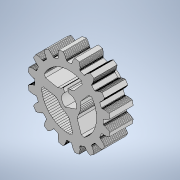
# Autodesk Inventor part: Ведущая шестерня дифференециала
Saved by Autodesk Inventor 2020 (Build 240168000, 168)
## iProperties
Created: 2021-05-23
Part Number: Ведущая шестерня дифференециала
Material: Типовые
Document SubType Name: Modeling
Designer: Антон
Density: 1 g/cm^3
Appearance: По умолчанию
Author: Антон
Autodesk Inventor part; units mm, degrees
(part 1 of 2)
ref_plane "YZ Plane" through (0, 0, 0) normal (1, 0, 0) x (0, 1, 0)
ref_plane "XZ Plane" through (0, 0, 0) normal (0, 1, 0) x (-1, 0, 0)
ref_plane "XY Plane" through (0, 0, 0) normal (0, 0, 1) x (1, 0, 0)
sketch "Эскиз1" plane through (0, 0, 0) normal (0, 0, 1) x (1, 0, 0)
  line L0 (1.5404, 9.3026) -> (1.5076, 9.387)
  line L1 (1.5076, 9.387) -> (1.4717, 9.4203)
  line L2 (1.4717, 9.4203) -> (1.4352, 9.4443)
  line L3 (1.4352, 9.4443) -> (1.3612, 9.4785)
  line L4 (1.3612, 9.4785) -> (1.2865, 9.5017)
  line L5 (1.2865, 9.5017) -> (1.2112, 9.5182)
  line L6 (1.2112, 9.5182) -> (1.0615, 9.5608)
  line L7 (1.0615, 9.5608) -> (0.9133, 9.6174)
  line L8 (0.9133, 9.6174) -> (0.7663, 9.6852)
  line L9 (0.7663, 9.6852) -> (0.6208, 9.7626)
  line L10 (0.6208, 9.7626) -> (0.4767, 9.8489)
  line L11 (0.4767, 9.8489) -> (0.3343, 9.9435)
  line L12 (0.3343, 9.9435) -> (0.1935, 10.0459)
  line L13 (0.1935, 10.0459) -> (0.0892, 10.1277)
  line L14 (0.0892, 10.1277) -> (0.2775, 11.074)
  line L15 (0.2775, 11.074) -> (0.4052, 11.1097)
  line L16 (0.4052, 11.1097) -> (0.5744, 11.1505)
  line L17 (0.5744, 11.1505) -> (0.7422, 11.1834)
  line L18 (0.7422, 11.1834) -> (0.9083, 11.208)
  line L19 (0.9083, 11.208) -> (1.0724, 11.2238)
  line L20 (1.0724, 11.2238) -> (1.2341, 11.2302)
  line L21 (1.2341, 11.2302) -> (1.3927, 11.2258)
  line L22 (1.3927, 11.2258) -> (1.5473, 11.2079)
  line L23 (1.5473, 11.2079) -> (1.6232, 11.1943)
  line L24 (1.6232, 11.1943) -> (1.7011, 11.1871)
  line L25 (1.7011, 11.1871) -> (1.7825, 11.1904)
  line L26 (1.7825, 11.1904) -> (1.8254, 11.1986)
  line L27 (1.8254, 11.1986) -> (1.8713, 11.2156)
  line L28 (1.8713, 11.2156) -> (1.9339, 11.281)
  line L29 (1.9339, 11.281) -> (2.2631, 12.0757)
  line L30 (2.2631, 12.0757) -> (2.2651, 12.1663)
  line L31 (2.2651, 12.1663) -> (2.2447, 12.2108)
  line L32 (2.2447, 12.2108) -> (2.2201, 12.247)
  line L33 (2.2201, 12.247) -> (2.1649, 12.3068)
  line L34 (2.1649, 12.3068) -> (2.1047, 12.3569)
  line L35 (2.1047, 12.3569) -> (2.0415, 12.4009)
  line L36 (2.0415, 12.4009) -> (1.9195, 12.4975)
  line L37 (1.9195, 12.4975) -> (1.8042, 12.6066)
  line L38 (1.8042, 12.6066) -> (1.6944, 12.7254)
  line L39 (1.6944, 12.7254) -> (1.5896, 12.8527)
  line L40 (1.5896, 12.8527) -> (1.4895, 12.9875)
  line L41 (1.4895, 12.9875) -> (1.3941, 13.1294)
  line L42 (1.3941, 13.1294) -> (1.3032, 13.2779)
  line L43 (1.3032, 13.2779) -> (1.2382, 13.3934)
  line L44 (1.2382, 13.3934) -> (1.7742, 14.1957)
  line L45 (1.7742, 14.1957) -> (1.9058, 14.1797)
  line L46 (1.9058, 14.1797) -> (2.0778, 14.1527)
  line L47 (2.0778, 14.1527) -> (2.2454, 14.1188)
  line L48 (2.2454, 14.1188) -> (2.4083, 14.078)
  line L49 (2.4083, 14.078) -> (2.5659, 14.0298)
  line L50 (2.5659, 14.0298) -> (2.7177, 13.9738)
  line L51 (2.7177, 13.9738) -> (2.8626, 13.909)
  line L52 (2.8626, 13.909) -> (2.9986, 13.8333)
  line L53 (2.9986, 13.8333) -> (3.0635, 13.7917)
  line L54 (3.0635, 13.7917) -> (3.1327, 13.7553)
  line L55 (3.1327, 13.7553) -> (3.2092, 13.7272)
  line L56 (3.2092, 13.7272) -> (3.2519, 13.7183)
  line L57 (3.2519, 13.7183) -> (3.3009, 13.7165)
  line L58 (3.3009, 13.7165) -> (3.3838, 13.753)
  line L59 (3.3838, 13.753) -> (3.9921, 14.3612)
  line L60 (3.9921, 14.3612) -> (4.0285, 14.4441)
  line L61 (4.0285, 14.4441) -> (4.0267, 14.4931)
  line L62 (4.0267, 14.4931) -> (4.0179, 14.5359)
  line L63 (4.0179, 14.5359) -> (3.9898, 14.6123)
  line L64 (3.9898, 14.6123) -> (3.9533, 14.6815)
  line L65 (3.9533, 14.6815) -> (3.9117, 14.7464)
  line L66 (3.9117, 14.7464) -> (3.836, 14.8824)
  line L67 (3.836, 14.8824) -> (3.7712, 15.0273)
  line L68 (3.7712, 15.0273) -> (3.7152, 15.1791)
  line L69 (3.7152, 15.1791) -> (3.6671, 15.3368)
  line L70 (3.6671, 15.3368) -> (3.6262, 15.4996)
  line L71 (3.6262, 15.4996) -> (3.5924, 15.6672)
  line L72 (3.5924, 15.6672) -> (3.5653, 15.8392)
  line L73 (3.5653, 15.8392) -> (3.5494, 15.9708)
  line L74 (3.5494, 15.9708) -> (4.3516, 16.5068)
  line L75 (4.3516, 16.5068) -> (4.4671, 16.4418)
  line L76 (4.4671, 16.4418) -> (4.6156, 16.351)
  line L77 (4.6156, 16.351) -> (4.7575, 16.2555)
  line L78 (4.7575, 16.2555) -> (4.8924, 16.1555)
  line L79 (4.8924, 16.1555) -> (5.0196, 16.0506)
  line L80 (5.0196, 16.0506) -> (5.1384, 15.9408)
  line L81 (5.1384, 15.9408) -> (5.2475, 15.8255)
  line L82 (5.2475, 15.8255) -> (5.3441, 15.7035)
  line L83 (5.3441, 15.7035) -> (5.3882, 15.6403)
  line L84 (5.3882, 15.6403) -> (5.4382, 15.5801)
  line L85 (5.4382, 15.5801) -> (5.4981, 15.5249)
  line L86 (5.4981, 15.5249) -> (5.5342, 15.5004)
  line L87 (5.5342, 15.5004) -> (5.5787, 15.4799)
  line L88 (5.5787, 15.4799) -> (5.6693, 15.4819)
  line L89 (5.6693, 15.4819) -> (6.464, 15.8111)
  line L90 (6.464, 15.8111) -> (6.5294, 15.8737)
  line L91 (6.5294, 15.8737) -> (6.5464, 15.9196)
  line L92 (6.5464, 15.9196) -> (6.5547, 15.9626)
  line L93 (6.5547, 15.9626) -> (6.5579, 16.0439)
  line L94 (6.5579, 16.0439) -> (6.5508, 16.1219)
  line L95 (6.5508, 16.1219) -> (6.5372, 16.1977)
  line L96 (6.5372, 16.1977) -> (6.5193, 16.3523)
  line L97 (6.5193, 16.3523) -> (6.5149, 16.511)
  line L98 (6.5149, 16.511) -> (6.5212, 16.6726)
  line L99 (6.5212, 16.6726) -> (6.5371, 16.8367)
  line L100 (6.5371, 16.8367) -> (6.5617, 17.0028)
  line L101 (6.5617, 17.0028) -> (6.5945, 17.1706)
  line L102 (6.5945, 17.1706) -> (6.6353, 17.3399)
  line L103 (6.6353, 17.3399) -> (6.671, 17.4675)
  line L104 (6.671, 17.4675) -> (7.6173, 17.6558)
  line L105 (7.6173, 17.6558) -> (7.6991, 17.5515)
  line L106 (7.6991, 17.5515) -> (7.8015, 17.4107)
  line L107 (7.8015, 17.4107) -> (7.8961, 17.2683)
  line L108 (7.8961, 17.2683) -> (7.9824, 17.1242)
  line L109 (7.9824, 17.1242) -> (8.0598, 16.9787)
  line L110 (8.0598, 16.9787) -> (8.1276, 16.8317)
  line L111 (8.1276, 16.8317) -> (8.1842, 16.6835)
  line L112 (8.1842, 16.6835) -> (8.2268, 16.5338)
  line L113 (8.2268, 16.5338) -> (8.2433, 16.4585)
  line L114 (8.2433, 16.4585) -> (8.2665, 16.3838)
  line L115 (8.2665, 16.3838) -> (8.3007, 16.3099)
  line L116 (8.3007, 16.3099) -> (8.3247, 16.2734)
  line L117 (8.3247, 16.2734) -> (8.358, 16.2375)
  line L118 (8.358, 16.2375) -> (8.4424, 16.2046)
  line L119 (8.4424, 16.2046) -> (9.3026, 16.2046)
  line L120 (9.3026, 16.2046) -> (9.387, 16.2375)
  line L121 (9.387, 16.2375) -> (9.4203, 16.2734)
  line L122 (9.4203, 16.2734) -> (9.4443, 16.3099)
  line L123 (9.4443, 16.3099) -> (9.4785, 16.3838)
  line L124 (9.4785, 16.3838) -> (9.5017, 16.4585)
  line L125 (9.5017, 16.4585) -> (9.5182, 16.5338)
  line L126 (9.5182, 16.5338) -> (9.5608, 16.6835)
  line L127 (9.5608, 16.6835) -> (9.6174, 16.8317)
  line L128 (9.6174, 16.8317) -> (9.6852, 16.9787)
  line L129 (9.6852, 16.9787) -> (9.7626, 17.1242)
  line L130 (9.7626, 17.1242) -> (9.8489, 17.2683)
  line L131 (9.8489, 17.2683) -> (9.9435, 17.4107)
  line L132 (9.9435, 17.4107) -> (10.0459, 17.5515)
  line L133 (10.0459, 17.5515) -> (10.1277, 17.6558)
  line L134 (10.1277, 17.6558) -> (11.074, 17.4675)
  line L135 (11.074, 17.4675) -> (11.1097, 17.3399)
  line L136 (11.1097, 17.3399) -> (11.1505, 17.1706)
  line L137 (11.1505, 17.1706) -> (11.1834, 17.0028)
  line L138 (11.1834, 17.0028) -> (11.208, 16.8367)
  line L139 (11.208, 16.8367) -> (11.2238, 16.6726)
  line L140 (11.2238, 16.6726) -> (11.2302, 16.511)
  line L141 (11.2302, 16.511) -> (11.2258, 16.3523)
  line L142 (11.2258, 16.3523) -> (11.2079, 16.1977)
  line L143 (11.2079, 16.1977) -> (11.1943, 16.1219)
  line L144 (11.1943, 16.1219) -> (11.1871, 16.0439)
  line L145 (11.1871, 16.0439) -> (11.1904, 15.9626)
  line L146 (11.1904, 15.9626) -> (11.1986, 15.9196)
  line L147 (11.1986, 15.9196) -> (11.2156, 15.8737)
  line L148 (11.2156, 15.8737) -> (11.281, 15.8111)
  line L149 (11.281, 15.8111) -> (12.0757, 15.4819)
  line L150 (12.0757, 15.4819) -> (12.1663, 15.4799)
  line L151 (12.1663, 15.4799) -> (12.2108, 15.5004)
  line L152 (12.2108, 15.5004) -> (12.247, 15.5249)
  line L153 (12.247, 15.5249) -> (12.3068, 15.5801)
  line L154 (12.3068, 15.5801) -> (12.3569, 15.6403)
  line L155 (12.3569, 15.6403) -> (12.4009, 15.7035)
  line L156 (12.4009, 15.7035) -> (12.4975, 15.8255)
  line L157 (12.4975, 15.8255) -> (12.6066, 15.9408)
  line L158 (12.6066, 15.9408) -> (12.7254, 16.0506)
  line L159 (12.7254, 16.0506) -> (12.8527, 16.1555)
  line L160 (12.8527, 16.1555) -> (12.9875, 16.2555)
  line L161 (12.9875, 16.2555) -> (13.1294, 16.351)
  line L162 (13.1294, 16.351) -> (13.2779, 16.4418)
  line L163 (13.2779, 16.4418) -> (13.3934, 16.5068)
  line L164 (13.3934, 16.5068) -> (14.1957, 15.9708)
  line L165 (14.1957, 15.9708) -> (14.1797, 15.8392)
  line L166 (14.1797, 15.8392) -> (14.1527, 15.6672)
  line L167 (14.1527, 15.6672) -> (14.1188, 15.4996)
  line L168 (14.1188, 15.4996) -> (14.078, 15.3368)
  line L169 (14.078, 15.3368) -> (14.0298, 15.1791)
  line L170 (14.0298, 15.1791) -> (13.9738, 15.0273)
  line L171 (13.9738, 15.0273) -> (13.909, 14.8824)
  line L172 (13.909, 14.8824) -> (13.8333, 14.7464)
  line L173 (13.8333, 14.7464) -> (13.7917, 14.6815)
  line L174 (13.7917, 14.6815) -> (13.7553, 14.6123)
  line L175 (13.7553, 14.6123) -> (13.7272, 14.5359)
  line L176 (13.7272, 14.5359) -> (13.7183, 14.4931)
  line L177 (13.7183, 14.4931) -> (13.7165, 14.4441)
  line L178 (13.7165, 14.4441) -> (13.753, 14.3612)
  line L179 (13.753, 14.3612) -> (14.3612, 13.753)
  line L180 (14.3612, 13.753) -> (14.4441, 13.7165)
  line L181 (14.4441, 13.7165) -> (14.4931, 13.7183)
  line L182 (14.4931, 13.7183) -> (14.5359, 13.7272)
  line L183 (14.5359, 13.7272) -> (14.6123, 13.7553)
  line L184 (14.6123, 13.7553) -> (14.6815, 13.7917)
  line L185 (14.6815, 13.7917) -> (14.7464, 13.8333)
  line L186 (14.7464, 13.8333) -> (14.8824, 13.909)
  line L187 (14.8824, 13.909) -> (15.0273, 13.9738)
  line L188 (15.0273, 13.9738) -> (15.1791, 14.0298)
  line L189 (15.1791, 14.0298) -> (15.3368, 14.078)
  line L190 (15.3368, 14.078) -> (15.4996, 14.1188)
  line L191 (15.4996, 14.1188) -> (15.6672, 14.1527)
  line L192 (15.6672, 14.1527) -> (15.8392, 14.1797)
  line L193 (15.8392, 14.1797) -> (15.9708, 14.1957)
  line L194 (15.9708, 14.1957) -> (16.5068, 13.3934)
  line L195 (16.5068, 13.3934) -> (16.4418, 13.2779)
  line L196 (16.4418, 13.2779) -> (16.351, 13.1294)
  line L197 (16.351, 13.1294) -> (16.2555, 12.9875)
  line L198 (16.2555, 12.9875) -> (16.1555, 12.8527)
  line L199 (16.1555, 12.8527) -> (16.0506, 12.7254)
  line L200 (16.0506, 12.7254) -> (15.9408, 12.6066)
  line L201 (15.9408, 12.6066) -> (15.8255, 12.4975)
  line L202 (15.8255, 12.4975) -> (15.7035, 12.4009)
  line L203 (15.7035, 12.4009) -> (15.6403, 12.3569)
  line L204 (15.6403, 12.3569) -> (15.5801, 12.3068)
  line L205 (15.5801, 12.3068) -> (15.5249, 12.247)
  line L206 (15.5249, 12.247) -> (15.5004, 12.2108)
  line L207 (15.5004, 12.2108) -> (15.4799, 12.1663)
  line L208 (15.4799, 12.1663) -> (15.4819, 12.0757)
  line L209 (15.4819, 12.0757) -> (15.8111, 11.281)
  line L210 (15.8111, 11.281) -> (15.8737, 11.2156)
  line L211 (15.8737, 11.2156) -> (15.9196, 11.1986)
  line L212 (15.9196, 11.1986) -> (15.9626, 11.1904)
  line L213 (15.9626, 11.1904) -> (16.0439, 11.1871)
  line L214 (16.0439, 11.1871) -> (16.1219, 11.1943)
  line L215 (16.1219, 11.1943) -> (16.1977, 11.2079)
  line L216 (16.1977, 11.2079) -> (16.3523, 11.2258)
  line L217 (16.3523, 11.2258) -> (16.511, 11.2302)
  line L218 (16.511, 11.2302) -> (16.6726, 11.2238)
  line L219 (16.6726, 11.2238) -> (16.8367, 11.208)
  line L220 (16.8367, 11.208) -> (17.0028, 11.1834)
  line L221 (17.0028, 11.1834) -> (17.1706, 11.1505)
  line L222 (17.1706, 11.1505) -> (17.3399, 11.1097)
  line L223 (17.3399, 11.1097) -> (17.4675, 11.074)
  line L224 (17.4675, 11.074) -> (17.6558, 10.1277)
  line L225 (17.6558, 10.1277) -> (17.5515, 10.0459)
  line L226 (17.5515, 10.0459) -> (17.4107, 9.9435)
  line L227 (17.4107, 9.9435) -> (17.2683, 9.8489)
  line L228 (17.2683, 9.8489) -> (17.1242, 9.7626)
  line L229 (17.1242, 9.7626) -> (16.9787, 9.6852)
  line L230 (16.9787, 9.6852) -> (16.8317, 9.6174)
  line L231 (16.8317, 9.6174) -> (16.6835, 9.5608)
  line L232 (16.6835, 9.5608) -> (16.5338, 9.5182)
  line L233 (16.5338, 9.5182) -> (16.4585, 9.5017)
  line L234 (16.4585, 9.5017) -> (16.3838, 9.4785)
  line L235 (16.3838, 9.4785) -> (16.3099, 9.4443)
  line L236 (16.3099, 9.4443) -> (16.2734, 9.4203)
  line L237 (16.2734, 9.4203) -> (16.2375, 9.387)
  line L238 (16.2375, 9.387) -> (16.2046, 9.3026)
  line L239 (16.2046, 9.3026) -> (16.2046, 8.4424)
  line L240 (16.2046, 8.4424) -> (16.2375, 8.358)
  line L241 (16.2375, 8.358) -> (16.2734, 8.3247)
  line L242 (16.2734, 8.3247) -> (16.3099, 8.3007)
  line L243 (16.3099, 8.3007) -> (16.3838, 8.2665)
  line L244 (16.3838, 8.2665) -> (16.4585, 8.2433)
  line L245 (16.4585, 8.2433) -> (16.5338, 8.2268)
  line L246 (16.5338, 8.2268) -> (16.6835, 8.1842)
  line L247 (16.6835, 8.1842) -> (16.8317, 8.1276)
  line L248 (16.8317, 8.1276) -> (16.9787, 8.0598)
  line L249 (16.9787, 8.0598) -> (17.1242, 7.9824)
  line L250 (17.1242, 7.9824) -> (17.2683, 7.8961)
  line L251 (17.2683, 7.8961) -> (17.4107, 7.8015)
  line L252 (17.4107, 7.8015) -> (17.5515, 7.6991)
  line L253 (17.5515, 7.6991) -> (17.6558, 7.6173)
  line L254 (17.6558, 7.6173) -> (17.4675, 6.671)
  line L255 (17.4675, 6.671) -> (17.3399, 6.6353)
  line L256 (17.3399, 6.6353) -> (17.1706, 6.5945)
  line L257 (17.1706, 6.5945) -> (17.0028, 6.5617)
  line L258 (17.0028, 6.5617) -> (16.8367, 6.5371)
  line L259 (16.8367, 6.5371) -> (16.6726, 6.5212)
  line L260 (16.6726, 6.5212) -> (16.511, 6.5149)
  line L261 (16.511, 6.5149) -> (16.3523, 6.5193)
  line L262 (16.3523, 6.5193) -> (16.1977, 6.5372)
  line L263 (16.1977, 6.5372) -> (16.1219, 6.5508)
  line L264 (16.1219, 6.5508) -> (16.0439, 6.5579)
  line L265 (16.0439, 6.5579) -> (15.9626, 6.5547)
  line L266 (15.9626, 6.5547) -> (15.9196, 6.5464)
  line L267 (15.9196, 6.5464) -> (15.8737, 6.5294)
  line L268 (15.8737, 6.5294) -> (15.8111, 6.464)
  line L269 (15.8111, 6.464) -> (15.4819, 5.6693)
  line L270 (15.4819, 5.6693) -> (15.4799, 5.5787)
  line L271 (15.4799, 5.5787) -> (15.5004, 5.5342)
  line L272 (15.5004, 5.5342) -> (15.5249, 5.4981)
  line L273 (15.5249, 5.4981) -> (15.5801, 5.4382)
  line L274 (15.5801, 5.4382) -> (15.6403, 5.3882)
  line L275 (15.6403, 5.3882) -> (15.7035, 5.3441)
  line L276 (15.7035, 5.3441) -> (15.8255, 5.2475)
  line L277 (15.8255, 5.2475) -> (15.9408, 5.1384)
  line L278 (15.9408, 5.1384) -> (16.0506, 5.0196)
  line L279 (16.0506, 5.0196) -> (16.1555, 4.8924)
  line L280 (16.1555, 4.8924) -> (16.2555, 4.7575)
  line L281 (16.2555, 4.7575) -> (16.351, 4.6156)
  line L282 (16.351, 4.6156) -> (16.4418, 4.4671)
  line L283 (16.4418, 4.4671) -> (16.5068, 4.3516)
  line L284 (16.5068, 4.3516) -> (15.9708, 3.5494)
  line L285 (15.9708, 3.5494) -> (15.8392, 3.5653)
  line L286 (15.8392, 3.5653) -> (15.6672, 3.5924)
  line L287 (15.6672, 3.5924) -> (15.4996, 3.6262)
  line L288 (15.4996, 3.6262) -> (15.3368, 3.6671)
  line L289 (15.3368, 3.6671) -> (15.1791, 3.7152)
  line L290 (15.1791, 3.7152) -> (15.0273, 3.7712)
  line L291 (15.0273, 3.7712) -> (14.8824, 3.836)
  line L292 (14.8824, 3.836) -> (14.7464, 3.9117)
  line L293 (14.7464, 3.9117) -> (14.6815, 3.9533)
  line L294 (14.6815, 3.9533) -> (14.6123, 3.9898)
  line L295 (14.6123, 3.9898) -> (14.5359, 4.0179)
  line L296 (14.5359, 4.0179) -> (14.4931, 4.0267)
  line L297 (14.4931, 4.0267) -> (14.4441, 4.0285)
  line L298 (14.4441, 4.0285) -> (14.3612, 3.9921)
  line L299 (14.3612, 3.9921) -> (13.753, 3.3838)
  line L300 (13.753, 3.3838) -> (13.7165, 3.3009)
  line L301 (13.7165, 3.3009) -> (13.7183, 3.2519)
  line L302 (13.7183, 3.2519) -> (13.7272, 3.2092)
  line L303 (13.7272, 3.2092) -> (13.7553, 3.1327)
  line L304 (13.7553, 3.1327) -> (13.7917, 3.0635)
  line L305 (13.7917, 3.0635) -> (13.8333, 2.9986)
  line L306 (13.8333, 2.9986) -> (13.909, 2.8626)
  line L307 (13.909, 2.8626) -> (13.9738, 2.7177)
  line L308 (13.9738, 2.7177) -> (14.0298, 2.5659)
  line L309 (14.0298, 2.5659) -> (14.078, 2.4083)
  line L310 (14.078, 2.4083) -> (14.1188, 2.2454)
  line L311 (14.1188, 2.2454) -> (14.1527, 2.0778)
  line L312 (14.1527, 2.0778) -> (14.1797, 1.9058)
  line L313 (14.1797, 1.9058) -> (14.1957, 1.7742)
  line L314 (14.1957, 1.7742) -> (13.3934, 1.2382)
  line L315 (13.3934, 1.2382) -> (13.2779, 1.3032)
  line L316 (13.2779, 1.3032) -> (13.1294, 1.3941)
  line L317 (13.1294, 1.3941) -> (12.9875, 1.4895)
  line L318 (12.9875, 1.4895) -> (12.8527, 1.5896)
  line L319 (12.8527, 1.5896) -> (12.7254, 1.6944)
  line L320 (12.7254, 1.6944) -> (12.6066, 1.8042)
  line L321 (12.6066, 1.8042) -> (12.4975, 1.9195)
  line L322 (12.4975, 1.9195) -> (12.4009, 2.0415)
  line L323 (12.4009, 2.0415) -> (12.3569, 2.1047)
  line L324 (12.3569, 2.1047) -> (12.3068, 2.1649)
  line L325 (12.3068, 2.1649) -> (12.247, 2.2201)
  line L326 (12.247, 2.2201) -> (12.2108, 2.2447)
  line L327 (12.2108, 2.2447) -> (12.1663, 2.2651)
  line L328 (12.1663, 2.2651) -> (12.0757, 2.2631)
  line L329 (12.0757, 2.2631) -> (11.281, 1.9339)
  line L330 (11.281, 1.9339) -> (11.2156, 1.8713)
  line L331 (11.2156, 1.8713) -> (11.1986, 1.8254)
  line L332 (11.1986, 1.8254) -> (11.1904, 1.7825)
  line L333 (11.1904, 1.7825) -> (11.1871, 1.7011)
  line L334 (11.1871, 1.7011) -> (11.1943, 1.6232)
  line L335 (11.1943, 1.6232) -> (11.2079, 1.5473)
  line L336 (11.2079, 1.5473) -> (11.2258, 1.3927)
  line L337 (11.2258, 1.3927) -> (11.2302, 1.2341)
  line L338 (11.2302, 1.2341) -> (11.2238, 1.0724)
  line L339 (11.2238, 1.0724) -> (11.208, 0.9083)
  line L340 (11.208, 0.9083) -> (11.1834, 0.7422)
  line L341 (11.1834, 0.7422) -> (11.1505, 0.5744)
  line L342 (11.1505, 0.5744) -> (11.1097, 0.4052)
  line L343 (11.1097, 0.4052) -> (11.074, 0.2775)
  line L344 (11.074, 0.2775) -> (10.1277, 0.0892)
  line L345 (10.1277, 0.0892) -> (10.0459, 0.1935)
  line L346 (10.0459, 0.1935) -> (9.9435, 0.3343)
  line L347 (9.9435, 0.3343) -> (9.8489, 0.4767)
  line L348 (9.8489, 0.4767) -> (9.7626, 0.6208)
  line L349 (9.7626, 0.6208) -> (9.6852, 0.7663)
  line L350 (9.6852, 0.7663) -> (9.6174, 0.9133)
  line L351 (9.6174, 0.9133) -> (9.5608, 1.0615)
  line L352 (9.5608, 1.0615) -> (9.5182, 1.2112)
  line L353 (9.5182, 1.2112) -> (9.5017, 1.2865)
  line L354 (9.5017, 1.2865) -> (9.4785, 1.3612)
  line L355 (9.4785, 1.3612) -> (9.4443, 1.4352)
  line L356 (9.4443, 1.4352) -> (9.4203, 1.4717)
  line L357 (9.4203, 1.4717) -> (9.387, 1.5076)
  line L358 (9.387, 1.5076) -> (9.3026, 1.5404)
  line L359 (9.3026, 1.5404) -> (8.4424, 1.5404)
  line L360 (8.4424, 1.5404) -> (8.358, 1.5076)
  line L361 (8.358, 1.5076) -> (8.3247, 1.4717)
  line L362 (8.3247, 1.4717) -> (8.3007, 1.4352)
  line L363 (8.3007, 1.4352) -> (8.2665, 1.3612)
  line L364 (8.2665, 1.3612) -> (8.2433, 1.2865)
  line L365 (8.2433, 1.2865) -> (8.2268, 1.2112)
  line L366 (8.2268, 1.2112) -> (8.1842, 1.0615)
  line L367 (8.1842, 1.0615) -> (8.1276, 0.9133)
  line L368 (8.1276, 0.9133) -> (8.0598, 0.7663)
  line L369 (8.0598, 0.7663) -> (7.9824, 0.6208)
  line L370 (7.9824, 0.6208) -> (7.8961, 0.4767)
  line L371 (7.8961, 0.4767) -> (7.8015, 0.3343)
  line L372 (7.8015, 0.3343) -> (7.6991, 0.1935)
  line L373 (7.6991, 0.1935) -> (7.6173, 0.0892)
  line L374 (7.6173, 0.0892) -> (6.671, 0.2775)
  line L375 (6.671, 0.2775) -> (6.6353, 0.4052)
  line L376 (6.6353, 0.4052) -> (6.5945, 0.5744)
  line L377 (6.5945, 0.5744) -> (6.5617, 0.7422)
  line L378 (6.5617, 0.7422) -> (6.5371, 0.9083)
  line L379 (6.5371, 0.9083) -> (6.5212, 1.0724)
  line L380 (6.5212, 1.0724) -> (6.5149, 1.2341)
  line L381 (6.5149, 1.2341) -> (6.5193, 1.3927)
  line L382 (6.5193, 1.3927) -> (6.5372, 1.5473)
  line L383 (6.5372, 1.5473) -> (6.5508, 1.6232)
  line L384 (6.5508, 1.6232) -> (6.5579, 1.7011)
  line L385 (6.5579, 1.7011) -> (6.5547, 1.7825)
  line L386 (6.5547, 1.7825) -> (6.5464, 1.8254)
  line L387 (6.5464, 1.8254) -> (6.5294, 1.8713)
  line L388 (6.5294, 1.8713) -> (6.464, 1.9339)
  line L389 (6.464, 1.9339) -> (5.6693, 2.2631)
  line L390 (5.6693, 2.2631) -> (5.5787, 2.2651)
  line L391 (5.5787, 2.2651) -> (5.5342, 2.2447)
  line L392 (5.5342, 2.2447) -> (5.4981, 2.2201)
  line L393 (5.4981, 2.2201) -> (5.4382, 2.1649)
  line L394 (5.4382, 2.1649) -> (5.3882, 2.1047)
  line L395 (5.3882, 2.1047) -> (5.3441, 2.0415)
  line L396 (5.3441, 2.0415) -> (5.2475, 1.9195)
  line L397 (5.2475, 1.9195) -> (5.1384, 1.8042)
  line L398 (5.1384, 1.8042) -> (5.0196, 1.6944)
  line L399 (5.0196, 1.6944) -> (4.8924, 1.5896)
  line L400 (4.8924, 1.5896) -> (4.7575, 1.4895)
  line L401 (4.7575, 1.4895) -> (4.6156, 1.3941)
  line L402 (4.6156, 1.3941) -> (4.4671, 1.3032)
  line L403 (4.4671, 1.3032) -> (4.3516, 1.2382)
  line L404 (4.3516, 1.2382) -> (3.5494, 1.7742)
  line L405 (3.5494, 1.7742) -> (3.5653, 1.9058)
  line L406 (3.5653, 1.9058) -> (3.5924, 2.0778)
  line L407 (3.5924, 2.0778) -> (3.6262, 2.2454)
  line L408 (3.6262, 2.2454) -> (3.6671, 2.4083)
  line L409 (3.6671, 2.4083) -> (3.7152, 2.5659)
  line L410 (3.7152, 2.5659) -> (3.7712, 2.7177)
  line L411 (3.7712, 2.7177) -> (3.836, 2.8626)
  line L412 (3.836, 2.8626) -> (3.9117, 2.9986)
  line L413 (3.9117, 2.9986) -> (3.9533, 3.0635)
  line L414 (3.9533, 3.0635) -> (3.9898, 3.1327)
  line L415 (3.9898, 3.1327) -> (4.0179, 3.2092)
  line L416 (4.0179, 3.2092) -> (4.0267, 3.2519)
  line L417 (4.0267, 3.2519) -> (4.0285, 3.3009)
  line L418 (4.0285, 3.3009) -> (3.9921, 3.3838)
  line L419 (3.9921, 3.3838) -> (3.3838, 3.9921)
  line L420 (3.3838, 3.9921) -> (3.3009, 4.0285)
  line L421 (3.3009, 4.0285) -> (3.2519, 4.0267)
  line L422 (3.2519, 4.0267) -> (3.2092, 4.0179)
  line L423 (3.2092, 4.0179) -> (3.1327, 3.9898)
  line L424 (3.1327, 3.9898) -> (3.0635, 3.9533)
  line L425 (3.0635, 3.9533) -> (2.9986, 3.9117)
  line L426 (2.9986, 3.9117) -> (2.8626, 3.836)
  line L427 (2.8626, 3.836) -> (2.7177, 3.7712)
  line L428 (2.7177, 3.7712) -> (2.5659, 3.7152)
  line L429 (2.5659, 3.7152) -> (2.4083, 3.6671)
  line L430 (2.4083, 3.6671) -> (2.2454, 3.6262)
  line L431 (2.2454, 3.6262) -> (2.0778, 3.5924)
  line L432 (2.0778, 3.5924) -> (1.9058, 3.5653)
  line L433 (1.9058, 3.5653) -> (1.7742, 3.5494)
  line L434 (1.7742, 3.5494) -> (1.2382, 4.3516)
  line L435 (1.2382, 4.3516) -> (1.3032, 4.4671)
  line L436 (1.3032, 4.4671) -> (1.3941, 4.6156)
  line L437 (1.3941, 4.6156) -> (1.4895, 4.7575)
  line L438 (1.4895, 4.7575) -> (1.5896, 4.8924)
  line L439 (1.5896, 4.8924) -> (1.6944, 5.0196)
  line L440 (1.6944, 5.0196) -> (1.8042, 5.1384)
  line L441 (1.8042, 5.1384) -> (1.9195, 5.2475)
  line L442 (1.9195, 5.2475) -> (2.0415, 5.3441)
  line L443 (2.0415, 5.3441) -> (2.1047, 5.3882)
  line L444 (2.1047, 5.3882) -> (2.1649, 5.4382)
  line L445 (2.1649, 5.4382) -> (2.2201, 5.4981)
  line L446 (2.2201, 5.4981) -> (2.2447, 5.5342)
  line L447 (2.2447, 5.5342) -> (2.2651, 5.5787)
  line L448 (2.2651, 5.5787) -> (2.2631, 5.6693)
  line L449 (2.2631, 5.6693) -> (1.9339, 6.464)
  line L450 (1.9339, 6.464) -> (1.8713, 6.5294)
  line L451 (1.8713, 6.5294) -> (1.8254, 6.5464)
  line L452 (1.8254, 6.5464) -> (1.7825, 6.5547)
  line L453 (1.7825, 6.5547) -> (1.7011, 6.5579)
  line L454 (1.7011, 6.5579) -> (1.6232, 6.5508)
  line L455 (1.6232, 6.5508) -> (1.5473, 6.5372)
  line L456 (1.5473, 6.5372) -> (1.3927, 6.5193)
  line L457 (1.3927, 6.5193) -> (1.2341, 6.5149)
  line L458 (1.2341, 6.5149) -> (1.0724, 6.5212)
  line L459 (1.0724, 6.5212) -> (0.9083, 6.5371)
  line L460 (0.9083, 6.5371) -> (0.7422, 6.5617)
  line L461 (0.7422, 6.5617) -> (0.5744, 6.5945)
  line L462 (0.5744, 6.5945) -> (0.4052, 6.6353)
  line L463 (0.4052, 6.6353) -> (0.2775, 6.671)
  line L464 (0.2775, 6.671) -> (0.0892, 7.6173)
  line L465 (0.0892, 7.6173) -> (0.1935, 7.6991)
  line L466 (0.1935, 7.6991) -> (0.3343, 7.8015)
  line L467 (0.3343, 7.8015) -> (0.4767, 7.8961)
  line L468 (0.4767, 7.8961) -> (0.6208, 7.9824)
  line L469 (0.6208, 7.9824) -> (0.7663, 8.0598)
  line L470 (0.7663, 8.0598) -> (0.9133, 8.1276)
  line L471 (0.9133, 8.1276) -> (1.0615, 8.1842)
  line L472 (1.0615, 8.1842) -> (1.2112, 8.2268)
  line L473 (1.2112, 8.2268) -> (1.2865, 8.2433)
  line L474 (1.2865, 8.2433) -> (1.3612, 8.2665)
  line L475 (1.3612, 8.2665) -> (1.4352, 8.3007)
  line L476 (1.4352, 8.3007) -> (1.4717, 8.3247)
  line L477 (1.4717, 8.3247) -> (1.5076, 8.358)
  line L478 (1.5076, 8.358) -> (1.5404, 8.4424)
  line L479 (1.5404, 8.4424) -> (1.5404, 9.3026)
  line L480 (6.047, 8.4605) -> (3.4326, 8.9806)
  line L481 (3.4326, 8.9806) -> (2.9676, 8.5861)
  line L482 (2.9676, 8.5861) -> (3, 8.1922)
  line L483 (3, 8.1922) -> (3.0586, 7.8013)
  line L484 (3.0586, 7.8013) -> (3.1431, 7.4153)
  line L485 (3.1431, 7.4153) -> (3.2533, 7.0357)
  line L486 (3.2533, 7.0357) -> (3.3886, 6.6644)
  line L487 (3.3886, 6.6644) -> (3.5484, 6.3029)
  line L488 (3.5484, 6.3029) -> (3.732, 5.9529)
  line L489 (3.732, 5.9529) -> (3.9385, 5.616)
  line L490 (3.9385, 5.616) -> (4.1671, 5.2936)
  line L491 (4.1671, 5.2936) -> (4.4168, 4.9872)
  line L492 (4.4168, 4.9872) -> (4.6863, 4.6982)
  line L493 (4.6863, 4.6982) -> (4.9746, 4.4278)
  line L494 (4.9746, 4.4278) -> (5.2803, 4.1773)
  line L495 (5.2803, 4.1773) -> (5.602, 3.9478)
  line L496 (5.602, 3.9478) -> (5.9384, 3.7402)
  line L497 (5.9384, 3.7402) -> (6.2878, 3.5557)
  line L498 (6.2878, 3.5557) -> (6.6489, 3.3949)
  line L499 (6.6489, 3.3949) -> (7.0198, 3.2585)
  line L500 (7.0198, 3.2585) -> (7.3991, 3.1473)
  line L501 (7.3991, 3.1473) -> (7.7849, 3.0616)
  line L502 (7.7849, 3.0616) -> (8.1756, 3.0019)
  line L503 (8.1756, 3.0019) -> (8.5694, 2.9685)
  line L504 (8.5694, 2.9685) -> (8.9645, 2.9614)
  line L505 (8.9645, 2.9614) -> (9.3593, 2.9808)
  line L506 (9.3593, 2.9808) -> (9.6897, 3.4932)
  line L507 (9.6897, 3.4932) -> (8.8329, 6.0174)
  line L508 (8.8329, 6.0174) -> (8.1387, 6.5764)
  line L509 (8.1387, 6.5764) -> (7.8323, 6.698)
  line L510 (7.8323, 6.698) -> (7.5453, 6.8602)
  line L511 (7.5453, 6.8602) -> (7.2831, 7.0602)
  line L512 (7.2831, 7.0602) -> (7.0507, 7.294)
  line L513 (7.0507, 7.294) -> (6.8523, 7.5573)
  line L514 (6.8523, 7.5573) -> (6.6918, 7.8453)
  line L515 (6.6918, 7.8453) -> (6.047, 8.4605)
  line L516 (10.642, 6.6316) -> (11.4989, 4.1074)
  line L517 (11.4989, 4.1074) -> (12.073, 3.902)
  line L518 (12.073, 3.902) -> (12.3979, 4.1269)
  line L519 (12.3979, 4.1269) -> (12.7072, 4.3731)
  line L520 (12.7072, 4.3731) -> (12.9992, 4.6393)
  line L521 (12.9992, 4.6393) -> (13.2728, 4.9245)
  line L522 (13.2728, 4.9245) -> (13.5268, 5.2274)
  line L523 (13.5268, 5.2274) -> (13.7599, 5.5465)
  line L524 (13.7599, 5.5465) -> (13.9712, 5.8805)
  line L525 (13.9712, 5.8805) -> (14.1598, 6.2278)
  line L526 (14.1598, 6.2278) -> (14.3246, 6.587)
  line L527 (14.3246, 6.587) -> (14.4652, 6.9564)
  line L528 (14.4652, 6.9564) -> (14.5807, 7.3343)
  line L529 (14.5807, 7.3343) -> (14.6707, 7.7192)
  line L530 (14.6707, 7.7192) -> (14.7348, 8.1092)
  line L531 (14.7348, 8.1092) -> (14.7727, 8.5025)
  line L532 (14.7727, 8.5025) -> (14.7843, 8.8976)
  line L533 (14.7843, 8.8976) -> (14.7694, 9.2925)
  line L534 (14.7694, 9.2925) -> (14.7281, 9.6856)
  line L535 (14.7281, 9.6856) -> (14.6607, 10.075)
  line L536 (14.6607, 10.075) -> (14.5674, 10.4591)
  line L537 (14.5674, 10.4591) -> (14.4487, 10.836)
  line L538 (14.4487, 10.836) -> (14.305, 11.2042)
  line L539 (14.305, 11.2042) -> (14.1371, 11.562)
  line L540 (14.1371, 11.562) -> (13.9457, 11.9077)
  line L541 (13.9457, 11.9077) -> (13.7315, 12.2399)
  line L542 (13.7315, 12.2399) -> (13.1225, 12.2699)
  line L543 (13.1225, 12.2699) -> (11.3649, 10.2657)
  line L544 (11.3649, 10.2657) -> (11.2279, 9.3851)
  line L545 (11.2279, 9.3851) -> (11.2758, 9.0589)
  line L546 (11.2758, 9.0589) -> (11.2788, 8.7292)
  line L547 (11.2788, 8.7292) -> (11.2367, 8.4022)
  line L548 (11.2367, 8.4022) -> (11.1505, 8.084)
  line L549 (11.1505, 8.084) -> (11.0216, 7.7806)
  line L550 (11.0216, 7.7806) -> (10.8525, 7.4976)
  line L551 (10.8525, 7.4976) -> (10.642, 6.6316)
  line L552 (9.9285, 11.5254) -> (11.6861, 13.5296)
  line L553 (11.6861, 13.5296) -> (11.5769, 14.1295)
  line L554 (11.5769, 14.1295) -> (11.2196, 14.2984)
  line L555 (11.2196, 14.2984) -> (10.8518, 14.4431)
  line L556 (10.8518, 14.4431) -> (10.4752, 14.5629)
  line L557 (10.4752, 14.5629) -> (10.0914, 14.6573)
  line L558 (10.0914, 14.6573) -> (9.7022, 14.7258)
  line L559 (9.7022, 14.7258) -> (9.3092, 14.7682)
  line L560 (9.3092, 14.7682) -> (8.9143, 14.7842)
  line L561 (8.9143, 14.7842) -> (8.5192, 14.7737)
  line L562 (8.5192, 14.7737) -> (8.1258, 14.737)
  line L563 (8.1258, 14.737) -> (7.7356, 14.6739)
  line L564 (7.7356, 14.6739) -> (7.3505, 14.585)
  line L565 (7.3505, 14.585) -> (6.9722, 14.4706)
  line L566 (6.9722, 14.4706) -> (6.6024, 14.3311)
  line L567 (6.6024, 14.3311) -> (6.2428, 14.1672)
  line L568 (6.2428, 14.1672) -> (5.8949, 13.9797)
  line L569 (5.8949, 13.9797) -> (5.5603, 13.7693)
  line L570 (5.5603, 13.7693) -> (5.2405, 13.5371)
  line L571 (5.2405, 13.5371) -> (4.937, 13.284)
  line L572 (4.937, 13.284) -> (4.651, 13.0112)
  line L573 (4.651, 13.0112) -> (4.3839, 12.7199)
  line L574 (4.3839, 12.7199) -> (4.1369, 12.4114)
  line L575 (4.1369, 12.4114) -> (3.911, 12.0871)
  line L576 (3.911, 12.0871) -> (3.7074, 11.7484)
  line L577 (3.7074, 11.7484) -> (3.5268, 11.3968)
  line L578 (3.5268, 11.3968) -> (3.8053, 10.8544)
  line L579 (3.8053, 10.8544) -> (6.4197, 10.3344)
  line L580 (6.4197, 10.3344) -> (7.2509, 10.6561)
  line L581 (7.2509, 10.6561) -> (7.5094, 10.8606)
  line L582 (7.5094, 10.8606) -> (7.7934, 11.0281)
  line L583 (7.7934, 11.0281) -> (8.0977, 11.1551)
  line L584 (8.0977, 11.1551) -> (8.4164, 11.2395)
  line L585 (8.4164, 11.2395) -> (8.7436, 11.2796)
  line L586 (8.7436, 11.2796) -> (9.0733, 11.2747)
  line L587 (9.0733, 11.2747) -> (9.9285, 11.5254)
  circle A0 centre (8.8725, 8.8725) radius 0.5
  line L588 (5.915, 8.8725) -> (11.83, 8.8725)
  line L589 (8.8725, 5.915) -> (8.8725, 11.83)
  point P0 (0, 0)
  constraints: 1180 end point, 1 centre point
extrude "Выдавливание1" add sketch "Эскиз1" along normal blind 5
sketch "Эскиз2" plane through (0, 0, 5) normal (0, 0, 1) x (1, 0, 0)
  circle A0 centre (8.8725, 8.8725) radius 0.5 projected
  circle A1 centre (8.8725, 8.8725) radius 1.6
  line L0 (7.036, 9.3051) -> (7.6789, 7.4113)
  line L1 (7.6789, 7.4113) -> (10.709, 8.4399)
  line L2 (10.709, 8.4399) -> (10.0662, 10.3337)
  line L3 (10.0662, 10.3337) -> (7.036, 9.3051)
  line L4 (7.036, 9.3051) -> (10.709, 8.4399) construction
  line L5 (7.6789, 7.4113) -> (10.0662, 10.3337) construction
  line L6 (8.0977, 11.1551) -> (7.7934, 11.0281) projected
  line L7 (8.4164, 11.2395) -> (8.0977, 11.1551) projected
  line L8 (7.6242, 10.9944) -> (8.5711, 11.3159)
  line L9 (8.5711, 11.3159) -> (9.0245, 9.9802)
  line L10 (9.0245, 9.9802) -> (8.0776, 9.6587)
  line L11 (8.0776, 9.6587) -> (7.6242, 10.9944)
  point P0 (0, 0)
  point P1 (8.5511, 9.8194)
  point P2 (8.8574, 10.4724)
  point P3 (7.9105, 10.151)
  point P4 (8.0112, 7.5241)
  point P5 (10.3767, 8.3271)
  dimension "d2" = 3.2
  dimension "d3" = 2
  dimension "d6" = 1
  constraints: 20 end point, 5 midpoint, 4 parallel, 3 perpendicular, 1 centre point, 1 coincident, 1 tangent
  measures "d2" diameter of A1
  measures "d3" distance of L2.end L1.end
  measures "d6" distance of L9.end L10.end
extrude "Выдавливание2" cut sketch "Эскиз2" against normal through all contours A1 L1 L3 | L3 L9 A1 | L9 L3 L11 A1 | A1 L11 L8 L9 | L11 L3 A1
sketch "Эскиз3" plane through (0, 0, 0) normal (0, 0, -1) x (-1, 0, 0)
  line L0 (-8.8574, 10.4724) -> (-8.5898, 11.2608)
  line L1 (-8.7436, 11.2796) -> (-8.5898, 11.2608)
  line L2 (-9.0733, 11.2747) -> (-8.7436, 11.2796)
  line L3 (-9.9285, 11.5254) -> (-9.0733, 11.2747)
  line L4 (-11.6861, 13.5296) -> (-9.9285, 11.5254)
  line L5 (-11.5769, 14.1295) -> (-11.6861, 13.5296)
  line L6 (-11.2196, 14.2984) -> (-11.5769, 14.1295)
  line L7 (-10.8518, 14.4431) -> (-11.2196, 14.2984)
  line L8 (-10.4752, 14.5629) -> (-10.8518, 14.4431)
  line L9 (-10.0914, 14.6573) -> (-10.4752, 14.5629)
  line L10 (-9.7022, 14.7258) -> (-10.0914, 14.6573)
  line L11 (-9.3092, 14.7682) -> (-9.7022, 14.7258)
  line L12 (-8.9143, 14.7842) -> (-9.3092, 14.7682)
  line L13 (-8.5192, 14.7737) -> (-8.9143, 14.7842)
  line L14 (-8.1258, 14.737) -> (-8.5192, 14.7737)
  line L15 (-7.7356, 14.6739) -> (-8.1258, 14.737)
  line L16 (-7.3505, 14.585) -> (-7.7356, 14.6739)
  line L17 (-6.9722, 14.4706) -> (-7.3505, 14.585)
  line L18 (-6.6024, 14.3311) -> (-6.9722, 14.4706)
  line L19 (-6.2428, 14.1672) -> (-6.6024, 14.3311)
  line L20 (-5.8949, 13.9797) -> (-6.2428, 14.1672)
  line L21 (-5.5603, 13.7693) -> (-5.8949, 13.9797)
  line L22 (-5.2405, 13.5371) -> (-5.5603, 13.7693)
  line L23 (-4.937, 13.284) -> (-5.2405, 13.5371)
  line L24 (-4.651, 13.0112) -> (-4.937, 13.284)
  line L25 (-4.3839, 12.7199) -> (-4.651, 13.0112)
  line L26 (-4.1369, 12.4114) -> (-4.3839, 12.7199)
  line L27 (-3.911, 12.0871) -> (-4.1369, 12.4114)
  line L28 (-3.7074, 11.7484) -> (-3.911, 12.0871)
  line L29 (-3.5268, 11.3968) -> (-3.7074, 11.7484)
  line L30 (-3.8053, 10.8544) -> (-3.5268, 11.3968)
  line L31 (-6.4197, 10.3344) -> (-3.8053, 10.8544)
  line L32 (-7.2509, 10.6561) -> (-6.4197, 10.3344)
  line L33 (-7.5094, 10.8606) -> (-7.2509, 10.6561)
  line L34 (-7.6429, 10.9393) -> (-7.5094, 10.8606)
  line L35 (-7.6429, 10.9393) -> (-7.9105, 10.151)
  arc A0 (-8.0112, 7.5241) -> (-7.9105, 10.151) centre (-8.8725, 8.8725) ccw
  line L36 (-8.0112, 7.5241) -> (-10.3767, 8.3271)
  arc A1 (-8.8574, 10.4724) -> (-10.3767, 8.3271) centre (-8.8725, 8.8725) ccw
  line L37 (-11.208, 16.8367) -> (-11.1834, 17.0028)
  line L38 (-11.2238, 16.6726) -> (-11.208, 16.8367)
  line L39 (-11.2302, 16.511) -> (-11.2238, 16.6726)
  line L40 (-11.2258, 16.3523) -> (-11.2302, 16.511)
  line L41 (-11.2079, 16.1977) -> (-11.2258, 16.3523)
  line L42 (-11.1943, 16.1219) -> (-11.2079, 16.1977)
  line L43 (-11.1871, 16.0439) -> (-11.1943, 16.1219)
  line L44 (-11.1904, 15.9626) -> (-11.1871, 16.0439)
  line L45 (-11.1986, 15.9196) -> (-11.1904, 15.9626)
  line L46 (-11.2156, 15.8737) -> (-11.1986, 15.9196)
  line L47 (-11.281, 15.8111) -> (-11.2156, 15.8737)
  line L48 (-12.0757, 15.4819) -> (-11.281, 15.8111)
  line L49 (-12.1663, 15.4799) -> (-12.0757, 15.4819)
  line L50 (-12.2108, 15.5004) -> (-12.1663, 15.4799)
  line L51 (-12.247, 15.5249) -> (-12.2108, 15.5004)
  line L52 (-12.3068, 15.5801) -> (-12.247, 15.5249)
  line L53 (-12.3569, 15.6403) -> (-12.3068, 15.5801)
  line L54 (-12.4009, 15.7035) -> (-12.3569, 15.6403)
  line L55 (-12.4975, 15.8255) -> (-12.4009, 15.7035)
  line L56 (-12.6066, 15.9408) -> (-12.4975, 15.8255)
  line L57 (-12.7254, 16.0506) -> (-12.6066, 15.9408)
  line L58 (-12.8527, 16.1555) -> (-12.7254, 16.0506)
  line L59 (-12.9875, 16.2555) -> (-12.8527, 16.1555)
  line L60 (-13.1294, 16.351) -> (-12.9875, 16.2555)
  line L61 (-13.2779, 16.4418) -> (-13.1294, 16.351)
  line L62 (-13.3934, 16.5068) -> (-13.2779, 16.4418)
  line L63 (-14.1957, 15.9708) -> (-13.3934, 16.5068)
  line L64 (-14.1797, 15.8392) -> (-14.1957, 15.9708)
  line L65 (-14.1527, 15.6672) -> (-14.1797, 15.8392)
  line L66 (-14.1188, 15.4996) -> (-14.1527, 15.6672)
  line L67 (-14.078, 15.3368) -> (-14.1188, 15.4996)
  line L68 (-14.0298, 15.1791) -> (-14.078, 15.3368)
  line L69 (-13.9738, 15.0273) -> (-14.0298, 15.1791)
  line L70 (-13.909, 14.8824) -> (-13.9738, 15.0273)
  line L71 (-13.8333, 14.7464) -> (-13.909, 14.8824)
  line L72 (-13.7917, 14.6815) -> (-13.8333, 14.7464)
  line L73 (-13.7553, 14.6123) -> (-13.7917, 14.6815)
  line L74 (-13.7272, 14.5359) -> (-13.7553, 14.6123)
  line L75 (-13.7183, 14.4931) -> (-13.7272, 14.5359)
  line L76 (-13.7165, 14.4441) -> (-13.7183, 14.4931)
  line L77 (-13.753, 14.3612) -> (-13.7165, 14.4441)
  line L78 (-14.3612, 13.753) -> (-13.753, 14.3612)
  line L79 (-14.4441, 13.7165) -> (-14.3612, 13.753)
  line L80 (-14.4931, 13.7183) -> (-14.4441, 13.7165)
  line L81 (-14.5359, 13.7272) -> (-14.4931, 13.7183)
  line L82 (-14.6123, 13.7553) -> (-14.5359, 13.7272)
  line L83 (-14.6815, 13.7917) -> (-14.6123, 13.7553)
  line L84 (-14.7464, 13.8333) -> (-14.6815, 13.7917)
  line L85 (-14.8824, 13.909) -> (-14.7464, 13.8333)
  line L86 (-15.0273, 13.9738) -> (-14.8824, 13.909)
  line L87 (-15.1791, 14.0298) -> (-15.0273, 13.9738)
  line L88 (-15.3368, 14.078) -> (-15.1791, 14.0298)
  line L89 (-15.4996, 14.1188) -> (-15.3368, 14.078)
  line L90 (-15.6672, 14.1527) -> (-15.4996, 14.1188)
  line L91 (-15.8392, 14.1797) -> (-15.6672, 14.1527)
  line L92 (-15.9708, 14.1957) -> (-15.8392, 14.1797)
  line L93 (-16.5068, 13.3934) -> (-15.9708, 14.1957)
  line L94 (-16.4418, 13.2779) -> (-16.5068, 13.3934)
  line L95 (-16.351, 13.1294) -> (-16.4418, 13.2779)
  line L96 (-16.2555, 12.9875) -> (-16.351, 13.1294)
  line L97 (-16.1555, 12.8527) -> (-16.2555, 12.9875)
  line L98 (-16.0506, 12.7254) -> (-16.1555, 12.8527)
  line L99 (-15.9408, 12.6066) -> (-16.0506, 12.7254)
  line L100 (-15.8255, 12.4975) -> (-15.9408, 12.6066)
  line L101 (-15.7035, 12.4009) -> (-15.8255, 12.4975)
  line L102 (-15.6403, 12.3569) -> (-15.7035, 12.4009)
  line L103 (-15.5801, 12.3068) -> (-15.6403, 12.3569)
  line L104 (-15.5249, 12.247) -> (-15.5801, 12.3068)
  line L105 (-15.5004, 12.2108) -> (-15.5249, 12.247)
  line L106 (-15.4799, 12.1663) -> (-15.5004, 12.2108)
  line L107 (-15.4819, 12.0757) -> (-15.4799, 12.1663)
  line L108 (-15.8111, 11.281) -> (-15.4819, 12.0757)
  line L109 (-15.8737, 11.2156) -> (-15.8111, 11.281)
  line L110 (-15.9196, 11.1986) -> (-15.8737, 11.2156)
  line L111 (-15.9626, 11.1904) -> (-15.9196, 11.1986)
  line L112 (-16.0439, 11.1871) -> (-15.9626, 11.1904)
  line L113 (-16.1219, 11.1943) -> (-16.0439, 11.1871)
  line L114 (-16.1977, 11.2079) -> (-16.1219, 11.1943)
  line L115 (-16.3523, 11.2258) -> (-16.1977, 11.2079)
  line L116 (-16.511, 11.2302) -> (-16.3523, 11.2258)
  line L117 (-16.6726, 11.2238) -> (-16.511, 11.2302)
  line L118 (-16.8367, 11.208) -> (-16.6726, 11.2238)
  line L119 (-17.0028, 11.1834) -> (-16.8367, 11.208)
  line L120 (-17.1706, 11.1505) -> (-17.0028, 11.1834)
  line L121 (-17.3399, 11.1097) -> (-17.1706, 11.1505)
  line L122 (-17.4675, 11.074) -> (-17.3399, 11.1097)
  line L123 (-17.6558, 10.1277) -> (-17.4675, 11.074)
  line L124 (-17.5515, 10.0459) -> (-17.6558, 10.1277)
  line L125 (-17.4107, 9.9435) -> (-17.5515, 10.0459)
  line L126 (-17.2683, 9.8489) -> (-17.4107, 9.9435)
  line L127 (-17.1242, 9.7626) -> (-17.2683, 9.8489)
  line L128 (-16.9787, 9.6852) -> (-17.1242, 9.7626)
  line L129 (-16.8317, 9.6174) -> (-16.9787, 9.6852)
  line L130 (-16.6835, 9.5608) -> (-16.8317, 9.6174)
  line L131 (-16.5338, 9.5182) -> (-16.6835, 9.5608)
  line L132 (-16.4585, 9.5017) -> (-16.5338, 9.5182)
  line L133 (-16.3838, 9.4785) -> (-16.4585, 9.5017)
  line L134 (-16.3099, 9.4443) -> (-16.3838, 9.4785)
  line L135 (-16.2734, 9.4203) -> (-16.3099, 9.4443)
  line L136 (-16.2375, 9.387) -> (-16.2734, 9.4203)
  line L137 (-16.2046, 9.3026) -> (-16.2375, 9.387)
  line L138 (-16.2046, 8.4424) -> (-16.2046, 9.3026)
  line L139 (-16.2375, 8.358) -> (-16.2046, 8.4424)
  line L140 (-16.2734, 8.3247) -> (-16.2375, 8.358)
  line L141 (-16.3099, 8.3007) -> (-16.2734, 8.3247)
  line L142 (-16.3838, 8.2665) -> (-16.3099, 8.3007)
  line L143 (-16.4585, 8.2433) -> (-16.3838, 8.2665)
  line L144 (-16.5338, 8.2268) -> (-16.4585, 8.2433)
  line L145 (-16.6835, 8.1842) -> (-16.5338, 8.2268)
  line L146 (-16.8317, 8.1276) -> (-16.6835, 8.1842)
  line L147 (-16.9787, 8.0598) -> (-16.8317, 8.1276)
  line L148 (-17.1242, 7.9824) -> (-16.9787, 8.0598)
  line L149 (-17.2683, 7.8961) -> (-17.1242, 7.9824)
  line L150 (-17.4107, 7.8015) -> (-17.2683, 7.8961)
  line L151 (-17.5515, 7.6991) -> (-17.4107, 7.8015)
  line L152 (-17.6558, 7.6173) -> (-17.5515, 7.6991)
  line L153 (-17.4675, 6.671) -> (-17.6558, 7.6173)
  line L154 (-17.3399, 6.6353) -> (-17.4675, 6.671)
  line L155 (-17.1706, 6.5945) -> (-17.3399, 6.6353)
  line L156 (-17.0028, 6.5617) -> (-17.1706, 6.5945)
  line L157 (-16.8367, 6.5371) -> (-17.0028, 6.5617)
  line L158 (-16.6726, 6.5212) -> (-16.8367, 6.5371)
  line L159 (-16.511, 6.5149) -> (-16.6726, 6.5212)
  line L160 (-16.3523, 6.5193) -> (-16.511, 6.5149)
  line L161 (-16.1977, 6.5372) -> (-16.3523, 6.5193)
  line L162 (-16.1219, 6.5508) -> (-16.1977, 6.5372)
  line L163 (-16.0439, 6.5579) -> (-16.1219, 6.5508)
  line L164 (-15.9626, 6.5547) -> (-16.0439, 6.5579)
  line L165 (-15.9196, 6.5464) -> (-15.9626, 6.5547)
  line L166 (-15.8737, 6.5294) -> (-15.9196, 6.5464)
  line L167 (-15.8111, 6.464) -> (-15.8737, 6.5294)
  line L168 (-15.4819, 5.6693) -> (-15.8111, 6.464)
  line L169 (-15.4799, 5.5787) -> (-15.4819, 5.6693)
  line L170 (-15.5004, 5.5342) -> (-15.4799, 5.5787)
  line L171 (-15.5249, 5.4981) -> (-15.5004, 5.5342)
  line L172 (-15.5801, 5.4382) -> (-15.5249, 5.4981)
  line L173 (-15.6403, 5.3882) -> (-15.5801, 5.4382)
  line L174 (-15.7035, 5.3441) -> (-15.6403, 5.3882)
  line L175 (-15.8255, 5.2475) -> (-15.7035, 5.3441)
  line L176 (-15.9408, 5.1384) -> (-15.8255, 5.2475)
  line L177 (-16.0506, 5.0196) -> (-15.9408, 5.1384)
  line L178 (-16.1555, 4.8924) -> (-16.0506, 5.0196)
  line L179 (-16.2555, 4.7575) -> (-16.1555, 4.8924)
  line L180 (-16.351, 4.6156) -> (-16.2555, 4.7575)
  line L181 (-16.4418, 4.4671) -> (-16.351, 4.6156)
  line L182 (-16.5068, 4.3516) -> (-16.4418, 4.4671)
  line L183 (-15.9708, 3.5494) -> (-16.5068, 4.3516)
  line L184 (-15.8392, 3.5653) -> (-15.9708, 3.5494)
  line L185 (-15.6672, 3.5924) -> (-15.8392, 3.5653)
  line L186 (-15.4996, 3.6262) -> (-15.6672, 3.5924)
  line L187 (-15.3368, 3.6671) -> (-15.4996, 3.6262)
  line L188 (-15.1791, 3.7152) -> (-15.3368, 3.6671)
  line L189 (-15.0273, 3.7712) -> (-15.1791, 3.7152)
  line L190 (-14.8824, 3.836) -> (-15.0273, 3.7712)
  line L191 (-14.7464, 3.9117) -> (-14.8824, 3.836)
  line L192 (-14.6815, 3.9533) -> (-14.7464, 3.9117)
  line L193 (-14.6123, 3.9898) -> (-14.6815, 3.9533)
  line L194 (-14.5359, 4.0179) -> (-14.6123, 3.9898)
  line L195 (-14.4931, 4.0267) -> (-14.5359, 4.0179)
  line L196 (-14.4441, 4.0285) -> (-14.4931, 4.0267)
  line L197 (-14.3612, 3.9921) -> (-14.4441, 4.0285)
  line L198 (-13.753, 3.3838) -> (-14.3612, 3.9921)
  line L199 (-13.7165, 3.3009) -> (-13.753, 3.3838)
  line L200 (-13.7183, 3.2519) -> (-13.7165, 3.3009)
  line L201 (-13.7272, 3.2092) -> (-13.7183, 3.2519)
  line L202 (-13.7553, 3.1327) -> (-13.7272, 3.2092)
  line L203 (-13.7917, 3.0635) -> (-13.7553, 3.1327)
  line L204 (-13.8333, 2.9986) -> (-13.7917, 3.0635)
  line L205 (-13.909, 2.8626) -> (-13.8333, 2.9986)
  line L206 (-13.9738, 2.7177) -> (-13.909, 2.8626)
  line L207 (-14.0298, 2.5659) -> (-13.9738, 2.7177)
  line L208 (-14.078, 2.4083) -> (-14.0298, 2.5659)
  line L209 (-14.1188, 2.2454) -> (-14.078, 2.4083)
  line L210 (-14.1527, 2.0778) -> (-14.1188, 2.2454)
  line L211 (-14.1797, 1.9058) -> (-14.1527, 2.0778)
  line L212 (-14.1957, 1.7742) -> (-14.1797, 1.9058)
  line L213 (-13.3934, 1.2382) -> (-14.1957, 1.7742)
  line L214 (-13.2779, 1.3032) -> (-13.3934, 1.2382)
  line L215 (-13.1294, 1.3941) -> (-13.2779, 1.3032)
  line L216 (-12.9875, 1.4895) -> (-13.1294, 1.3941)
  line L217 (-12.8527, 1.5896) -> (-12.9875, 1.4895)
  line L218 (-12.7254, 1.6944) -> (-12.8527, 1.5896)
  line L219 (-12.6066, 1.8042) -> (-12.7254, 1.6944)
  line L220 (-12.4975, 1.9195) -> (-12.6066, 1.8042)
  line L221 (-12.4009, 2.0415) -> (-12.4975, 1.9195)
  line L222 (-12.3569, 2.1047) -> (-12.4009, 2.0415)
  line L223 (-12.3068, 2.1649) -> (-12.3569, 2.1047)
  line L224 (-12.247, 2.2201) -> (-12.3068, 2.1649)
  line L225 (-12.2108, 2.2447) -> (-12.247, 2.2201)
  line L226 (-12.1663, 2.2651) -> (-12.2108, 2.2447)
  line L227 (-12.0757, 2.2631) -> (-12.1663, 2.2651)
  line L228 (-11.281, 1.9339) -> (-12.0757, 2.2631)
  line L229 (-11.2156, 1.8713) -> (-11.281, 1.9339)
  line L230 (-11.1986, 1.8254) -> (-11.2156, 1.8713)
  line L231 (-11.1904, 1.7825) -> (-11.1986, 1.8254)
  line L232 (-11.1871, 1.7011) -> (-11.1904, 1.7825)
  line L233 (-11.1943, 1.6232) -> (-11.1871, 1.7011)
  line L234 (-11.2079, 1.5473) -> (-11.1943, 1.6232)
  line L235 (-11.2258, 1.3927) -> (-11.2079, 1.5473)
  line L236 (-11.2302, 1.2341) -> (-11.2258, 1.3927)
  line L237 (-11.2238, 1.0724) -> (-11.2302, 1.2341)
  line L238 (-11.208, 0.9083) -> (-11.2238, 1.0724)
  line L239 (-11.1834, 0.7422) -> (-11.208, 0.9083)
  line L240 (-11.1505, 0.5744) -> (-11.1834, 0.7422)
  line L241 (-11.1097, 0.4052) -> (-11.1505, 0.5744)
  line L242 (-11.074, 0.2775) -> (-11.1097, 0.4052)
  line L243 (-10.1277, 0.0892) -> (-11.074, 0.2775)
  line L244 (-10.0459, 0.1935) -> (-10.1277, 0.0892)
  line L245 (-9.9435, 0.3343) -> (-10.0459, 0.1935)
  line L246 (-9.8489, 0.4767) -> (-9.9435, 0.3343)
  line L247 (-9.7626, 0.6208) -> (-9.8489, 0.4767)
  line L248 (-9.6852, 0.7663) -> (-9.7626, 0.6208)
  line L249 (-9.6174, 0.9133) -> (-9.6852, 0.7663)
  line L250 (-9.5608, 1.0615) -> (-9.6174, 0.9133)
  line L251 (-9.5182, 1.2112) -> (-9.5608, 1.0615)
  line L252 (-9.5017, 1.2865) -> (-9.5182, 1.2112)
  line L253 (-9.4785, 1.3612) -> (-9.5017, 1.2865)
  line L254 (-9.4443, 1.4352) -> (-9.4785, 1.3612)
  line L255 (-9.4203, 1.4717) -> (-9.4443, 1.4352)
  line L256 (-9.387, 1.5076) -> (-9.4203, 1.4717)
  line L257 (-9.3026, 1.5404) -> (-9.387, 1.5076)
  line L258 (-8.4424, 1.5404) -> (-9.3026, 1.5404)
  line L259 (-8.358, 1.5076) -> (-8.4424, 1.5404)
  line L260 (-8.3247, 1.4717) -> (-8.358, 1.5076)
  line L261 (-8.3007, 1.4352) -> (-8.3247, 1.4717)
  line L262 (-8.2665, 1.3612) -> (-8.3007, 1.4352)
  line L263 (-8.2433, 1.2865) -> (-8.2665, 1.3612)
  line L264 (-8.2268, 1.2112) -> (-8.2433, 1.2865)
  line L265 (-8.1842, 1.0615) -> (-8.2268, 1.2112)
  line L266 (-8.1276, 0.9133) -> (-8.1842, 1.0615)
  line L267 (-8.0598, 0.7663) -> (-8.1276, 0.9133)
  line L268 (-7.9824, 0.6208) -> (-8.0598, 0.7663)
  line L269 (-7.8961, 0.4767) -> (-7.9824, 0.6208)
  line L270 (-7.8015, 0.3343) -> (-7.8961, 0.4767)
  line L271 (-7.6991, 0.1935) -> (-7.8015, 0.3343)
  line L272 (-7.6173, 0.0892) -> (-7.6991, 0.1935)
  line L273 (-6.671, 0.2775) -> (-7.6173, 0.0892)
  line L274 (-6.6353, 0.4052) -> (-6.671, 0.2775)
  line L275 (-6.5945, 0.5744) -> (-6.6353, 0.4052)
  line L276 (-6.5617, 0.7422) -> (-6.5945, 0.5744)
  line L277 (-6.5371, 0.9083) -> (-6.5617, 0.7422)
  line L278 (-6.5212, 1.0724) -> (-6.5371, 0.9083)
  line L279 (-6.5149, 1.2341) -> (-6.5212, 1.0724)
  line L280 (-6.5193, 1.3927) -> (-6.5149, 1.2341)
  line L281 (-6.5372, 1.5473) -> (-6.5193, 1.3927)
  line L282 (-6.5508, 1.6232) -> (-6.5372, 1.5473)
  line L283 (-6.5579, 1.7011) -> (-6.5508, 1.6232)
  line L284 (-6.5547, 1.7825) -> (-6.5579, 1.7011)
  line L285 (-6.5464, 1.8254) -> (-6.5547, 1.7825)
  line L286 (-6.5294, 1.8713) -> (-6.5464, 1.8254)
  line L287 (-6.464, 1.9339) -> (-6.5294, 1.8713)
  line L288 (-5.6693, 2.2631) -> (-6.464, 1.9339)
  line L289 (-5.5787, 2.2651) -> (-5.6693, 2.2631)
  line L290 (-5.5342, 2.2447) -> (-5.5787, 2.2651)
  line L291 (-5.4981, 2.2201) -> (-5.5342, 2.2447)
  line L292 (-5.4382, 2.1649) -> (-5.4981, 2.2201)
  line L293 (-5.3882, 2.1047) -> (-5.4382, 2.1649)
  line L294 (-5.3441, 2.0415) -> (-5.3882, 2.1047)
  line L295 (-5.2475, 1.9195) -> (-5.3441, 2.0415)
  line L296 (-5.1384, 1.8042) -> (-5.2475, 1.9195)
  line L297 (-5.0196, 1.6944) -> (-5.1384, 1.8042)
  line L298 (-4.8924, 1.5896) -> (-5.0196, 1.6944)
  line L299 (-4.7575, 1.4895) -> (-4.8924, 1.5896)
  line L300 (-4.6156, 1.3941) -> (-4.7575, 1.4895)
  line L301 (-4.4671, 1.3032) -> (-4.6156, 1.3941)
  line L302 (-4.3516, 1.2382) -> (-4.4671, 1.3032)
  line L303 (-3.5494, 1.7742) -> (-4.3516, 1.2382)
  line L304 (-3.5653, 1.9058) -> (-3.5494, 1.7742)
  line L305 (-3.5924, 2.0778) -> (-3.5653, 1.9058)
  line L306 (-3.6262, 2.2454) -> (-3.5924, 2.0778)
  line L307 (-3.6671, 2.4083) -> (-3.6262, 2.2454)
  line L308 (-3.7152, 2.5659) -> (-3.6671, 2.4083)
  line L309 (-3.7712, 2.7177) -> (-3.7152, 2.5659)
  line L310 (-3.836, 2.8626) -> (-3.7712, 2.7177)
  line L311 (-3.9117, 2.9986) -> (-3.836, 2.8626)
  line L312 (-3.9533, 3.0635) -> (-3.9117, 2.9986)
  line L313 (-3.9898, 3.1327) -> (-3.9533, 3.0635)
  line L314 (-4.0179, 3.2092) -> (-3.9898, 3.1327)
  line L315 (-4.0267, 3.2519) -> (-4.0179, 3.2092)
  line L316 (-4.0285, 3.3009) -> (-4.0267, 3.2519)
  line L317 (-3.9921, 3.3838) -> (-4.0285, 3.3009)
  line L318 (-3.3838, 3.9921) -> (-3.9921, 3.3838)
  line L319 (-3.3009, 4.0285) -> (-3.3838, 3.9921)
  line L320 (-3.2519, 4.0267) -> (-3.3009, 4.0285)
  line L321 (-3.2092, 4.0179) -> (-3.2519, 4.0267)
  line L322 (-3.1327, 3.9898) -> (-3.2092, 4.0179)
  line L323 (-3.0635, 3.9533) -> (-3.1327, 3.9898)
  line L324 (-2.9986, 3.9117) -> (-3.0635, 3.9533)
  line L325 (-2.8626, 3.836) -> (-2.9986, 3.9117)
  line L326 (-2.7177, 3.7712) -> (-2.8626, 3.836)
  line L327 (-2.5659, 3.7152) -> (-2.7177, 3.7712)
  line L328 (-2.4083, 3.6671) -> (-2.5659, 3.7152)
  line L329 (-2.2454, 3.6262) -> (-2.4083, 3.6671)
  line L330 (-2.0778, 3.5924) -> (-2.2454, 3.6262)
  line L331 (-1.9058, 3.5653) -> (-2.0778, 3.5924)
  line L332 (-1.7742, 3.5494) -> (-1.9058, 3.5653)
  line L333 (-1.2382, 4.3516) -> (-1.7742, 3.5494)
  line L334 (-1.3032, 4.4671) -> (-1.2382, 4.3516)
  line L335 (-1.3941, 4.6156) -> (-1.3032, 4.4671)
  line L336 (-1.4895, 4.7575) -> (-1.3941, 4.6156)
  line L337 (-1.5896, 4.8924) -> (-1.4895, 4.7575)
  line L338 (-1.6944, 5.0196) -> (-1.5896, 4.8924)
  line L339 (-1.8042, 5.1384) -> (-1.6944, 5.0196)